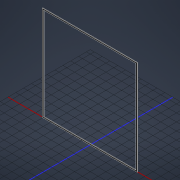
# Autodesk Inventor part: Foamtape Top
Saved by Autodesk Inventor 2022.2 (Build 262287010, 287A)
## iProperties
Created: 2022-03-16
Part Number: Foamtape Top
Material: Gummi, Silikon
Document SubType Name: Modeling
Designer: sleib
Density: 1.25 g/cm^3
Appearance: Gummi - Schwarz
Author: sleib
Autodesk Inventor part; units mm, degrees
ref_plane "YZ Plane" through (0, 0, 0) normal (1, 0, 0) x (0, 1, 0)
ref_plane "XZ Plane" through (0, 0, 0) normal (0, 1, 0) x (-1, 0, 0)
ref_plane "XY Plane" through (0, 0, 0) normal (0, 0, 1) x (1, 0, 0)
sketch "Skizze1" plane through (0, 0, 0) normal (0, 0, 1) x (1, 0, 0)
  line L0 (-242, -242) -> (242, -242)
  line L1 (242, -242) -> (242, 242)
  line L2 (242, 242) -> (-242, 242)
  line L3 (-242, 242) -> (-242, -242)
  line L4 (-242, -242) -> (242, 242) construction
  line L5 (242, -242) -> (-242, 242) construction
  line L6 (-236, 236) -> (236, 236)
  line L7 (236, 236) -> (236, -236)
  line L8 (236, -236) -> (-236, -236)
  line L9 (-236, -236) -> (-236, 236)
  point P0 (0, 0)
  dimension "d0" = 484
  dimension "d1" = 484
  dimension "d2" = 6
  constraints: 20 end point, 4 parallel, 2 midpoint, 2 perpendicular, 1 horizontal, 3 other
  measures "d0" distance of L2.end L1.end
  measures "d1" distance of L1.end L0.end
  measures "d2" distance between parallel lines of L2 L6
extrude "Extrusion1" add sketch "Skizze1" along normal blind 3
